# Autodesk Inventor part: Cylindrical Cam
Saved by Autodesk Inventor 2015 (Build 190159000, 159)
## iProperties
Created: 2015-04-20
Part Number: Cylindrical Cam
Material: Steel
Document SubType Name: Modeling
Designer: WASHHSST
Density: 7.85 g/cm^3
Appearance: Steel
CustomPartVersion: 1
Author: WASHHSST
Autodesk Inventor part; units mm, degrees
ref_plane "YZ Plane" through (0, 0, 0) normal (1, 0, 0) x (0, 1, 0)
ref_plane "Start Plane" through (0, 0, -88.9) normal (0, 0, 1) x (1, 0, 0)
sketch "Base Sketch" plane through (0, 0, -88.9) normal (0, 0, 1) x (1, 0, 0)
  circle A0 centre (0, 0) radius 88.9
  circle A1 centre (0, 0) radius 114.3
  dimension "d0" = 177.8
  dimension "d1" = 228.6
  constraints: 2 centre point, 2 coincident
  measures "d0" diameter of A0
  measures "d1" diameter of A1
extrude "Cam body" add sketch "Base Sketch" along normal blind 431.8
sketch3d "Path Sketch"
ref_plane "Profile Plane" through (0, 101.6, 0) normal (1, 0.0004, -0.0001) x (-0.0004, 1, 0)
sketch "Profile Sketch" plane through (0, 101.6, 0) normal (1, 0.0004, -0.0001) x (-0.0004, 1, 0)
  line L0 (17.78, -38.1) -> (-17.78, -38.1)
  point P0 (0, 0)
  dimension "d2" = 35.56
  dimension "d3" = 38.1
  dimension "d14" = 17.78
  constraints: 2 end point, 1 horizontal
  measures "d2" distance of L0.start L0.end
  measures "d3" distance from line of point (0, 0) L0
  measures "d14" horizontal distance of L0.end point (0, 0)
feature "End Surface" [suppressed]
feature "Split Body" [suppressed]
equation "\"d0\" = 2 * da_r0 - da_bv"
equation "\"d1\" = 2 * da_r0 + da_bv"
equation "\"d6\" = da_maxh - d9 + da_rk"
equation "\"d2\" = da_bv + 0.1 * da_r0"
equation "\"d3\" = da_rk"
equation "\"d14\" = 0.5 * da_bv + 0.05 * da_r0"
equation "\"da_bv\" = 25.4"
equation "\"da_r0\" = 101.6"
equation "\"da_rk\" = 38.1"
equation "\"da_maxh\" = 304.8"
equation "\"da_minh\" = 0"
equation "\"d9\" = -da_rk + da_minh - 0.5 * da_r0"
body "Solid1"
body "Srf1"
